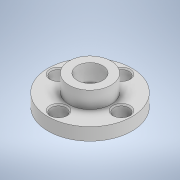
# Autodesk Inventor part: втулка
Saved by Autodesk Inventor 2021 (Build 250183000, 183)
## iProperties
Created: 2023-02-16
Part Number: втулка
Material: Типовые
Document SubType Name: Modeling
Designer: Tasya
Density: 1 g/cm^3
Appearance: По умолчанию
Author: Tasya
Autodesk Inventor part; units mm, degrees
ref_plane "YZ Plane" through (0, 0, 0) normal (1, 0, 0) x (0, 1, 0)
ref_plane "XZ Plane" through (0, 0, 0) normal (0, 1, 0) x (-1, 0, 0)
ref_plane "XY Plane" through (0, 0, 0) normal (0, 0, 1) x (1, 0, 0)
sketch "Эскиз1" plane through (0, 0, 0) normal (0, 1, 0) x (-1, 0, 0)
  circle A0 centre (0, 0) radius 10
  dimension "d0" = 20
  constraints: 1 centre point, 1 coincident
  measures "d0" diameter of A0
extrude "Выдавливание1" add sketch "Эскиз1" along normal blind 3
sketch "Эскиз2" plane through (0, 3, 0) normal (0, 1, 0) x (1, 0, 0)
  circle A0 centre (0, 0) radius 10 projected
  circle A1 centre (0, 0) radius 5
  dimension "d3" = 10
  constraints: 1 centre point, 1 coincident
  measures "d3" diameter of A1
extrude "Выдавливание2" add sketch "Эскиз2" along normal blind 4 contours A1
sketch "Эскиз3" plane through (0, 7, 0) normal (0, 1, 0) x (1, 0, 0)
  circle A0 centre (0, 0) radius 5 projected
  constraints: 1 coincident
hole "Отверстие1" at (0, 7, 0) direction (0, -1, 0) diameter 6.1 depth 4
sketch "Эскиз4" plane through (0, 3, 0) normal (0, 1, 0) x (1, 0, 0)
  circle A0 centre (0, 0) radius 5 projected
  circle A1 centre (0, 0) radius 10 projected
  circle A2 centre (0, 0) radius 7.5 construction
  point P0 (0, -7.5)
  dimension "d22" = 15
  dimension "d13" = 5
  constraints: 1 coincident, 1 vertical alignment, 2 other
  measures "d13" radial gap between concentric circles of A0 A1
hole "Отверстие2" at (0, 3, 7.5) direction (0, -1, 0) diameter 3.6 depth 4 countersink diameter 4.2 countersink angle 90
pattern_circular "Круговой массив1" count 4 over 360 about axis through (0, 5, 0) along (0, 1, 0) of "Отверстие2"
